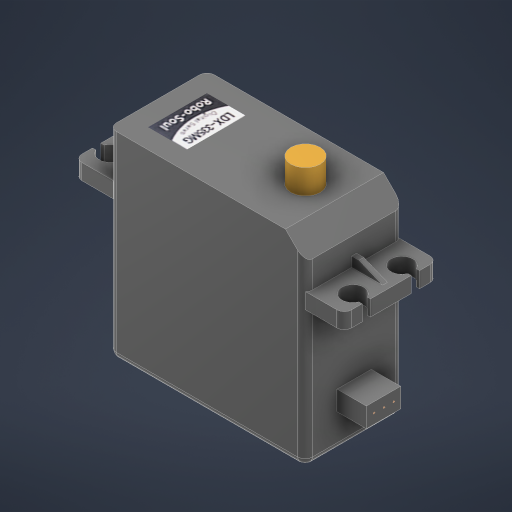
# Autodesk Inventor part: LDX-335MG_Servo_15kg_cm
Saved by Autodesk Inventor 2023 (Build 270158000, 158)
## iProperties
Created: 2023-02-24
Part Number: LDX-335MG_Servo_15kg_cm
Material: Steel
Document SubType Name: Modeling
Designer: roota
Density: 7.85 g/cm^3
Appearance: Smooth - Black
Mass: 265.715 g
Surface Area: 78.4173 cm^2
Volume: 33.849 cm^3
Author: roota
Autodesk Inventor part; units mm, degrees
ref_plane "YZ Plane" through (0, 0, 0) normal (1, 0, 0) x (0, 1, 0)
ref_plane "XY Plane" through (0, 0, 0) normal (0, 0, 1) x (1, 0, 0)
sketch "Sketch1" plane through (0, 0, 0) normal (0, 1, 0) x (-1, 0, 0)
  line L0 (30.1, 10) -> (-9.9, 10)
  line L1 (-9.9, 10) -> (-9.9, -10)
  line L2 (-9.9, -10) -> (30.1, -10)
  line L3 (30.1, -10) -> (30.1, 10)
  line L4 (30.1, 10) -> (-9.9, -10) construction
  line L5 (-9.9, 10) -> (30.1, -10) construction
  point P0 (0, 0)
  point P1 (10.1, 0)
  dimension "d0" = 40
  dimension "d1" = 20
  dimension "d2" = 9.9
  constraints: 12 end point, 2 midpoint, 2 parallel, 1 horizontal, 1 horizontal alignment, 1 perpendicular
  measures "d0" distance of L2.end L1.end
  measures "d1" distance of L1.end L0.end
  measures "d2" distance from line of point (0, 0) L1
extrude "Extrusion1" add sketch "Sketch1" along normal blind 40.5
ref_plane "Work Plane1" through (0, 27.8, 0) normal (0, 1, 0) x (-1, 0, 0)
sketch "Sketch2" plane through (0, 27.8, 0) normal (0, 1, 0) x (-1, 0, 0)
  line L0 (37.6, -9.5) -> (-17.4, -9.5)
  line L1 (-17.4, -9.5) -> (-17.4, 9.5)
  line L2 (-17.4, 9.5) -> (37.6, 9.5)
  line L3 (37.6, 9.5) -> (37.6, -9.5)
  circle A0 centre (-14.65, 5) radius 2.25
  circle A1 centre (-14.65, -5) radius 2.25
  circle A2 centre (34.85, -5) radius 2.25
  circle A3 centre (34.85, 5) radius 2.25
  line L4 (30.1, -10) -> (30.1, 10) projected
  line L5 (-9.9, 10) -> (-9.9, -10) projected
  line L6 (-17.9, -4.15) -> (-15.9, -4.15)
  line L7 (-15.9, -4.15) -> (-15.9, -5.85)
  line L8 (-15.9, -5.85) -> (-17.9, -5.85)
  line L9 (-17.9, -5.85) -> (-17.9, -4.15)
  line L10 (-17.9, -4.15) -> (-15.9, -5.85) construction
  line L11 (-15.9, -4.15) -> (-17.9, -5.85) construction
  line L12 (10.1, 11.9779) -> (10.1, -10.6791)
  line L13 (38.1, -4.15) -> (36.1, -4.15)
  line L14 (36.1, -4.15) -> (36.1, -5.85)
  line L15 (36.1, -5.85) -> (38.1, -5.85)
  line L16 (38.1, -5.85) -> (38.1, -4.15)
  line L17 (38.1, -4.15) -> (36.1, -5.85) construction
  line L18 (36.1, -4.15) -> (38.1, -5.85) construction
  line L19 (37.6, 0) -> (-17.4, 0)
  line L20 (-17.9, 4.15) -> (-15.9, 4.15)
  line L21 (-15.9, 4.15) -> (-15.9, 5.85)
  line L22 (-15.9, 5.85) -> (-17.9, 5.85)
  line L23 (-17.9, 5.85) -> (-17.9, 4.15)
  line L24 (-17.9, 4.15) -> (-15.9, 5.85) construction
  line L25 (-15.9, 4.15) -> (-17.9, 5.85) construction
  line L26 (36.1, 4.15) -> (36.1, 5.85)
  line L27 (38.1, 4.15) -> (36.1, 4.15)
  line L28 (36.1, 5.85) -> (38.1, 5.85)
  line L29 (38.1, 5.85) -> (38.1, 4.15)
  line L30 (38.1, 4.15) -> (36.1, 5.85) construction
  line L31 (36.1, 4.15) -> (38.1, 5.85) construction
  point P0 (0, 0)
  point P1 (-9.9, -9.5)
  point P2 (-9.9, 9.5)
  point P3 (-17.15, 6.1456)
  point P4 (-17.15, 3.8544)
  point P5 (-17.15, -3.8544)
  point P6 (-17.15, -6.1456)
  point P7 (30.1, 9.5)
  point P8 (30.1, -9.5)
  point P9 (37.35, -6.1456)
  point P10 (37.35, -3.8544)
  point P11 (37.35, 3.8544)
  point P12 (37.35, 6.1456)
  point P13 (-16.9, -5)
  point P14 (-15.9, -5)
  point P15 (37.1, -5)
  point P16 (36.1, -5)
  point P17 (-16.9, 5)
  point P18 (-15.9, 5)
  point P19 (36.1, 5)
  point P20 (37.1, 5)
  point P21 (-17.4, 5.85)
  point P22 (-16.7333, 5.85)
  point P23 (-16.7333, 4.15)
  point P24 (-17.4, 4.15)
  point P25 (-17.4, -4.15)
  point P26 (-16.7333, -4.15)
  point P27 (-16.7333, -5.85)
  point P28 (-17.4, -5.85)
  point P29 (37.6, -5.85)
  point P30 (36.9333, -5.85)
  point P31 (36.9333, -4.15)
  point P32 (37.6, -4.15)
  point P33 (37.6, 4.15)
  point P34 (36.9333, 4.15)
  point P35 (36.9333, 5.85)
  point P36 (37.6, 5.85)
  dimension "d6" = 19
  dimension "d7" = 9.5
  dimension "d8" = 55
  dimension "d9" = 4.5
  dimension "d10" = 49.5
  dimension "d11" = 10
  dimension "d12" = 2.75
  dimension "d13" = 5
  dimension "d14" = 7.5
  dimension "d15" = 7.5
  dimension "d59" = 1.7
  dimension "d60" = 2
  dimension "d61" = 49.5
  constraints: 60 end point, 20 symmetric about line, 5 midpoint, 4 parallel, 3 centre point, 3 horizontal alignment, 2 horizontal, 2 perpendicular, 2 vertical alignment, 1 equal radius, 1 vertical, 5 other
  measures "d6" distance of L0.end L1.end
  measures "d7" distance from line of point (0, 0) L2
  measures "d8" distance of L1.end L2.end
  measures "d9" diameter of A0
  measures "d10" distance of A0.centre A3.centre
  measures "d11" distance of point (-14.65, -5) A0.centre
  measures "d12" distance from line of L1 A0.centre
  measures "d13" vertical distance of point (0, 0) point (-14.65, -5)
  measures "d14" distance between parallel lines of L4 L3
  measures "d15" distance between parallel lines of L1 L5
  measures "d59" distance of L6.end L7.end
  measures "d60" distance of L6.start L6.end
  measures "d61" diameter of A3.centre L12
extrude "Extrusion2" add sketch "Sketch2" along normal blind 3.2 contours L0 L4 L19 L3 L13 A2 L15 | L0 L12 L19 L4 | L0 L5 L19 L12 | L19 L12 L2 L4 | L4 L2 L3 L28 A3 L27 L19 | L0 L1 L8 A1 L6 L19 L5 | L19 L5 L2 L12 | L19 L1 L20 A0 L22 L2 L5
chamfer "Chamfer1" distance 4 angle 45 1 edges at (9.9, 40.5, 0)
fillet "Fillet1" radius 1.5 12 edges at (-30.1, 20.25, 10) (-30.1, 20.25, -10) (9.9, 18.25, -10) (9.9, 18.25, 10) (17.4, 29.4, -9.5) (17.4, 29.4, 9.5) (-37.6, 29.4, 9.5) (-37.6, 29.4, -9.5) (-10.1, 0, 10) (-30.1, 0, 0) (-10.1, 0, -10) (9.9, 0, 0)
sketch "Sketch3" plane through (0, 40.5, 0) normal (0, 1, 0) x (1, 0, 0)
  circle A0 centre (0, 0) radius 3
  dimension "d19" = 6
  constraints: 1 centre point, 1 coincident
  measures "d19" diameter of A0
extrude "Extrusion3" add sketch "Sketch3" along normal blind 5
sketch "Sketch6" plane through (0, 0, 0) normal (0, 0, 1) x (1, 0, 0)
  line L0 (11.4, 33) -> (16.2, 31)
  line L1 (-31.6, 33) -> (-36.4, 31)
  line L2 (-29.718, 27.8) -> (-36.1, 27.8) projected
  line L3 (-31.6, 33) -> (-30.1, 33)
  line L4 (-37.6, 31) -> (-37.6, 27.8) projected
  line L5 (-36.1, 31) -> (-29.718, 31) projected
  line L6 (-30.1, 40.5) -> (-30.1, 31) projected
  line L7 (-10.1, 48.4931) -> (-10.1, 32.7483)
  line L8 (9.9, 31) -> (9.9, 36.5) projected
  line L9 (-30.1, 27.8) -> (-30.1, 1.5) projected
  line L10 (9.9, 1.5) -> (9.9, 27.8) projected
  line L11 (11.4, 33) -> (9.9, 33)
  line L12 (9.518, 31) -> (15.9, 31) projected
  point P0 (0, 0)
  dimension "d63" = 5.2
  dimension "d64" = 1.2
  dimension "d65" = 1.5
  dimension "d66" = 40
  dimension "d67" = 40
  constraints: 10 end point, 4 point on line, 2 horizontal, 1 vertical, 2 other
  measures "d63" distance from line of L1.start L2
  measures "d64" distance from line of L1.end L4
  measures "d65" distance of L1.start L3.end
  measures "d66" diameter of L6 L7
  measures "d67" distance between parallel lines of L9 L10
extrude "Rib1" add sketch "Sketch6" along normal mid plane 1 rib yes fills toward (-30.85, 32.95) open curves L3 L1
extrude "Rib2" add sketch "Sketch6" along normal mid plane 1 rib yes fills toward (10.65, 32.95) open curves L11 L0
sketch "Sketch7" plane through (9.9, 1.5, -8.5) normal (1, 0, 0) x (0, 0, -1)
  line L0 (0, 0) -> (-17, 0) projected
  line L1 (0, 26.3) -> (0, 0) projected
  line L2 (-17, 0) -> (0, 0)
  line L3 (0, 0) -> (0, 5.1466)
  line L4 (0, 5.1466) -> (-17, 5.1466)
  line L5 (-17, 5.1466) -> (-17, 0)
  line L6 (-12, 5.5) -> (-5, 5.5)
  line L7 (-5, 5.5) -> (-5, 9.5)
  line L8 (-5, 9.5) -> (-12, 9.5)
  line L9 (-12, 9.5) -> (-12, 5.5)
  line L10 (-12, 5.5) -> (-5, 9.5) construction
  line L11 (-5, 5.5) -> (-12, 9.5) construction
  line L12 (-17, -1.5) -> (0, -1.5) projected
  line L13 (-18.5, 36.5) -> (-18.5, 0) projected
  point P0 (-8.5, -1.5)
  point P1 (-8.5, 7.5)
  dimension "d68" = 7
  dimension "d69" = 4
  dimension "d70" = 7
  dimension "d71" = 10
  constraints: 20 end point, 4 parallel, 2 horizontal, 2 midpoint, 2 perpendicular, 1 point on line
  measures "d68" distance of L8.end L7.end
  measures "d69" distance of L7.end L6.end
  measures "d70" distance between parallel lines of L6 L12
  measures "d71" distance from line of L13 point (-8.5, 7.5)
extrude "Extrusion6" add sketch "Sketch7" along normal blind 6 contours L9 L8 L7 L6
sketch "Sketch8" plane through (0, 40.5, 0) normal (0, 1, 0) x (1, 0, 0)
  line L0 (-18.1937, 6) -> (-18.1937, -6) construction
  line L1 (-18.1937, -6) -> (-26.1, -6) construction
  line L2 (-26.1, -6) -> (-26.1, 6) construction
  line L3 (-26.1, 6) -> (-18.1937, 6) construction
  line L4 (5.9, 10) -> (-28.6, 10) projected
  line L5 (-28.6, -10) -> (5.9, -10) projected
  line L6 (-30.1, 8.5) -> (-30.1, -8.5) projected
  point P0 (0, 0)
  dimension "d50" = 4
  dimension "d51" = 4
  dimension "d52" = 4
  constraints: 2 other
  measures "d50" distance between parallel lines of L4 L3
  measures "d51" distance between parallel lines of L5 L1
  measures "d52" distance between parallel lines of L6 L2
decal "Decal1"
sketch "Sketch9" plane through (15.9, 1.5, -8.5) normal (1, 0, 0) x (0, 0, -1)
  line L0 (-10.5, 7.5) -> (-6.5, 7.5) construction
  line L1 (-12, 5.5) -> (-5, 5.5) projected
  point P0 (-8.5, -1.5)
  point P1 (-8.5, 7.5)
  dimension "d54" = 2
  dimension "d72" = 2
  constraints: 2 coincident, 2 end point, 1 horizontal, 1 midpoint, 1 vertical alignment
  measures "d54" distance of point (-8.5, 7.5) L0.end
  measures "d72" distance from line of point (-8.5, 7.5) L1
equation "\"d7\" = 0.5 * d6"
equation "\"d12\" = -0.5 * d10 + 0.5 * d8"
equation "\"d13\" = 0.5 * d11"
equation "\"d14\" = d15"
equation "\"d61\" = d10"
equation "\"d66\" = d67"
equation "\"d51\" = d50"
body "Solid1"
